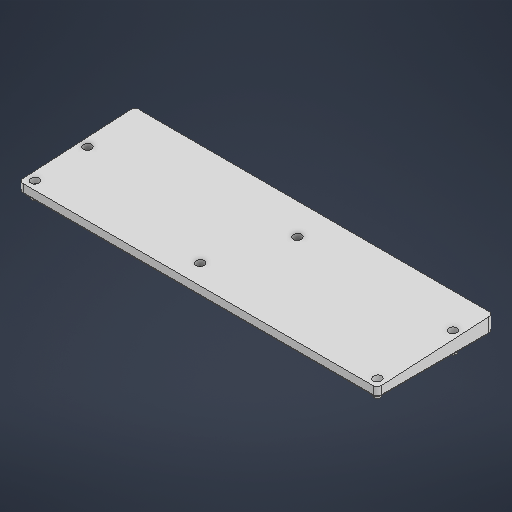
# Autodesk Inventor part: Bottom
Saved by Autodesk Inventor 2026 (Build 300175050, 175E)
## iProperties
Created: 2025-06-14
Part Number: Bottom
Material: Generisch
Document SubType Name: Modeling
Designer: nikla
Density: 1 g/cm^3
Appearance: Vorgabe
Author: nikla
Autodesk Inventor part; units mm, degrees
ref_plane "YZ Plane" through (0, 0, 0) normal (1, 0, 0) x (0, 1, 0)
ref_plane "XZ Plane" through (0, 0, 0) normal (0, 1, 0) x (-1, 0, 0)
sketch "Skizze1" plane through (0, 0, 0) normal (0, 0, 1) x (1, 0, 0)
  circle A0 centre (-271.1, -102.4) radius 2.25
  circle A1 centre (-271, -139.7) radius 2.25
  circle A2 centre (-140.5, -84.3) radius 2.25
  circle A3 centre (-161.5, -132.1) radius 2.25
  circle A4 centre (-28.4, -139.7) radius 2.25
  circle A5 centre (-28.2, -86.4) radius 2.25
  circle A6 centre (-216.6, -72.6) radius 2.25
  point P0 (0, 0)
extrude "Extrusion1" add sketch "Skizze1" along normal blind 3 contours A0 | A1 | A2 | A3 | A4 | A5
sketch "Skizze2" plane through (-216.6, -72.6, 3) normal (0, 0, 1) x (1, 0, 0)
  line L0 (-57.14, 7.74) -> (190.86, 7.74) projected
  arc A0 (192.36, 6.24) -> (190.86, 7.74) centre (190.86, 6.24) ccw projected
  line L1 (192.36, 6.24) -> (192.36, -69.76) projected
  arc A1 (190.86, -71.26) -> (192.36, -69.76) centre (190.86, -69.76) ccw projected
  line L2 (190.86, -71.26) -> (-57.14, -71.26) projected
  arc A2 (-58.64, -69.76) -> (-57.14, -71.26) centre (-57.14, -69.76) ccw projected
  line L3 (-58.64, -69.76) -> (-58.64, 6.24) projected
  arc A3 (-57.14, 7.74) -> (-58.64, 6.24) centre (-57.14, 6.24) ccw projected
  point P0 (216.6, 72.6)
ref_plane "Arbeitsebene1" through (-276.74, -145.36, 4.8625) normal (0, 0, 1) x (1, 0, 0)
extrude "Extrusion2" add sketch "Skizze2" along normal up to surface (1.8625 mm away)
sketch "Skizze3" plane through (-273.74, -143.86, 4.8625) normal (0, 0, 1) x (1, 0, 0)
  line L0 (248, 80.5) -> (0, 80.5) projected
  arc A0 (0, 80.5) -> (-3, 77.5) centre (0, 77.5) ccw projected
  line L1 (-3, 77.5) -> (-3, 1.5) projected
  arc A1 (-3, 1.5) -> (0, -1.5) centre (0, 1.5) ccw projected
  line L2 (0, -1.5) -> (248, -1.5) projected
  arc A2 (248, -1.5) -> (251, 1.5) centre (248, 1.5) ccw projected
  line L3 (251, 1.5) -> (251, 77.5) projected
  arc A3 (251, 77.5) -> (248, 80.5) centre (248, 77.5) ccw projected
  point P0 (273.74, 143.86)
extrude "Extrusion3" add sketch "Skizze3" along normal blind 5
sketch "Skizze4" plane through (-273.74, -143.86, 9.8625) normal (0, 0, 1) x (1, 0, 0)
  circle A0 centre (245.54, 57.46) radius 2.25 construction
  circle A1 centre (245.34, 4.16) radius 2.25 construction
  circle A2 centre (133.24, 59.56) radius 1.2295 projected
  circle A3 centre (133.24, 59.56) radius 1.2295 projected
  circle A4 centre (112.24, 11.76) radius 1.6 projected
  circle A5 centre (57.14, 71.26) radius 2.25 projected
  circle A6 centre (2.64, 41.46) radius 1.2295 projected
  circle A7 centre (2.74, 4.16) radius 1.2295 projected
  circle A8 centre (2.64, 41.46) radius 2.85
  circle A9 centre (2.74, 4.16) radius 2.85
  circle A10 centre (57.14, 71.26) radius 2.85
  circle A11 centre (112.24, 11.76) radius 2.25 projected
  circle A12 centre (112.24, 11.76) radius 2.85
  circle A13 centre (133.24, 59.56) radius 2.25 projected
  circle A14 centre (133.24, 59.56) radius 2.85
  circle A15 centre (245.54, 57.46) radius 2.85
  circle A16 centre (245.34, 4.16) radius 2.85
  point P0 (273.74, 143.86)
  dimension "d6" = 5.7
  dimension "d7" = 5.7
  dimension "d8" = 5.7
  dimension "d9" = 5.7
  dimension "d10" = 5.7
  dimension "d11" = 5.7
  dimension "d12" = 5.7
  constraints: 7 centre point, 7 coincident
  measures "d6" diameter of A8
  measures "d7" diameter of A9
  measures "d8" diameter of A10
  measures "d9" diameter of A12
  measures "d10" diameter of A14
  measures "d11" diameter of A15
  measures "d12" diameter of A16
extrude "Extrusion4" cut sketch "Skizze4" against normal blind 3.2 contours A2 | A4 | A6 | A7 | A8 | A9 | A11 | A12 | A13 | A14 | A15 | A16
sketch "Skizze5" plane through (-273.74, -143.86, 9.8625) normal (0, 0, 1) x (1, 0, 0)
  circle A0 centre (245.54, 57.46) radius 2.85 projected
  circle A1 centre (245.34, 4.16) radius 2.85 projected
  circle A2 centre (112.24, 11.76) radius 2.85 projected
  circle A3 centre (133.24, 59.56) radius 2.85 projected
  circle A4 centre (57.14, 71.26) radius 2.85 projected
  circle A5 centre (2.64, 41.46) radius 2.85 projected
  circle A6 centre (2.74, 4.16) radius 2.85 projected
  point P0 (273.74, 143.86)
hole "Bohrung1" at (-271, -139.7, 9.8625) at (-271.1, -102.4, 9.8625) at (-161.5, -132.1, 9.8625) at (-140.5, -84.3, 9.8625) at (-28.2, -86.4, 9.8625) at (-28.4, -139.7, 9.8625) direction (0, 0, -1) diameter 3.2 depth 23.862
sketch "Skizze6" plane through (-273.74, -143.86, 9.8625) normal (0, 0, 1) x (1, 0, 0)
  circle A0 centre (245.54, 57.46) radius 2.85 projected
  circle A1 centre (112.24, 11.76) radius 2.85 projected
  circle A2 centre (2.74, 4.16) radius 2.85 projected
  circle A3 centre (245.34, 4.16) radius 2.85 projected
  circle A4 centre (133.24, 59.56) radius 2.85 projected
  circle A5 centre (2.64, 41.46) radius 2.85 projected
  arc A6 (0, 80.5) -> (-3, 77.5) centre (0, 77.5) ccw projected
  line L0 (-3, 77.5) -> (-3, 1.5) projected
  arc A7 (-3, 1.5) -> (0, -1.5) centre (0, 1.5) ccw projected
  line L1 (0, -1.5) -> (248, -1.5) projected
  arc A8 (248, -1.5) -> (251, 1.5) centre (248, 1.5) ccw projected
  line L2 (251, 1.5) -> (251, 77.5) projected
  arc A9 (251, 77.5) -> (248, 80.5) centre (248, 77.5) ccw projected
  line L3 (248, 80.5) -> (0, 80.5) projected
  point P0 (273.74, 143.86)
extrude "Extrusion5" add sketch "Skizze6" along normal blind 5
sketch "Skizze7" plane through (-22.74, -142.36, 4.8625) normal (1, 0, 0) x (0, 0, -1)
  line L0 (-10, 0) -> (-10, 76) projected
  line L1 (-10, 0) -> (-10, -3) projected
  line L2 (0, -3) -> (-10, -3) projected
  line L3 (0, 79) -> (-10, 79) projected
  line L4 (-10, 79) -> (-10, 76) projected
  line L5 (-10, 79) -> (-5.5, -3)
  point P0 (4.8625, 142.36)
  dimension "d27" = 4.5
  constraints: 2 end point, 1 point on line
  measures "d27" distance of L5.end L1.end
extrude "Extrusion6" cut sketch "Skizze7" against normal through all
